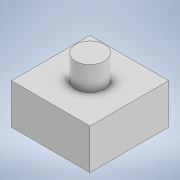
# Autodesk Inventor part: Pot
Saved by Autodesk Inventor 2022 (Build 260153000, 153)
## iProperties
Created: 2022-04-06
Part Number: Pot
Material: Generic
Document SubType Name: Modeling
Designer: awp
Density: 1 g/cm^3
Appearance: Default
Author: awp
Autodesk Inventor part; units mm, degrees
ref_plane "YZ Plane" through (0, 0, 0) normal (1, 0, 0) x (0, 1, 0)
ref_plane "XZ Plane" through (0, 0, 0) normal (0, 1, 0) x (-1, 0, 0)
ref_plane "XY Plane" through (0, 0, 0) normal (0, 0, 1) x (1, 0, 0)
sketch "Sketch1" plane through (0, 0, 0) normal (0, 1, 0) x (-1, 0, 0)
  line L0 (0, 0) -> (9.75, 0)
  line L1 (9.75, 0) -> (9.75, -9.75)
  line L2 (9.75, -9.75) -> (0, -9.75)
  line L3 (0, -9.75) -> (0, 0)
  dimension "d0" = 9.75
  dimension "d1" = 9.75
  constraints: 8 end point, 2 parallel, 1 horizontal, 1 perpendicular
  measures "d0" distance of L1.end L2.end
  measures "d1" distance of L0.end L1.end
extrude "Extrusion1" add sketch "Sketch1" along normal blind 5
sketch "Sketch2" plane through (0, 5, 0) normal (0, 1, 0) x (1, 0, 0)
  line L0 (0, 9.75) -> (-9.75, 9.75) projected
  line L1 (-9.75, 9.75) -> (-9.75, 0) projected
  line L2 (-9.75, 0) -> (0, 0) projected
  line L3 (0, 0) -> (0, 9.75) projected
  circle A0 centre (-4.875, 4.875) radius 1.8
  dimension "d4" = 3.6
  constraints: 1 centre point
  measures "d4" diameter of A0
extrude "Extrusion2" add sketch "Sketch2" along normal blind 3 contours A0
body "Solid1"
